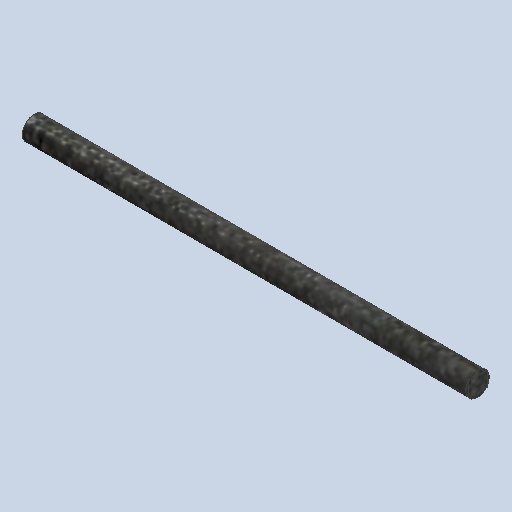
# Autodesk Inventor part: GuiderodsRS3
Saved by Autodesk Inventor 2024.3 (Build 283343000, 343)
## iProperties
Created: 2025-08-09
Part Number: GuiderodsRS3
Material: Steel
Document SubType Name: Modeling
Designer: ajclo
Density: 7.85 g/cm^3
Appearance: Plate
Mass: 14.4828 g
Surface Area: 15.1565 cm^2
Volume: 1.84494 cm^3
Author: ajclo
Autodesk Inventor part; units mm, degrees
ref_plane "YZ Plane" through (0, 0, 0) normal (1, 0, 0) x (0, 1, 0)
ref_plane "XZ Plane" through (0, 0, 0) normal (0, 1, 0) x (-1, 0, 0)
ref_plane "XY Plane" through (0, 0, 0) normal (0, 0, 1) x (1, 0, 0)
sketch "Sketch1" plane through (0, 0, 0) normal (1, 0, 0) x (0, 1, 0)
  circle A0 centre (0, 0) radius 2.5
  dimension "d0" = 5
  constraints: 1 centre point, 1 coincident
  measures "d0" diameter of A0
extrude "Extrusion1" add sketch "Sketch1" along normal blind 94
sketch "Sketch2" plane through (94, 0, 0) normal (1, 0, 0) x (0, 0, -1)
  circle A0 centre (0, 0) radius 2.5 projected
  line L0 (-1.955, 1.5582) -> (1.9325, 1.5582)
  line L1 (1.9325, 1.5582) -> (1.9325, -1.586)
  line L2 (1.9325, -1.586) -> (-1.955, -1.586)
  line L3 (-1.955, -1.586) -> (-1.955, 1.5582)
  point P0 (-1.955, -1.5582)
  point P1 (-1.9325, -1.586)
  constraints: 8 end point, 2 parallel, 2 point on circle, 1 horizontal, 1 perpendicular
extrude "Extrusion2" cut sketch "Sketch2" against normal blind 0.1 contours A0 L1 L0 | L3 A0 | A0 L2
body "Solid1"
